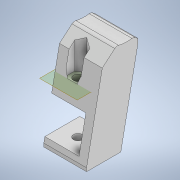
# Autodesk Inventor part: IntakeStop
Saved by Autodesk Inventor 2020 (Build 240168000, 168)
## iProperties
Created: 2020-02-14
Part Number: IntakeStop
Material: Generic
Document SubType Name: Modeling
Designer: srini
Density: 1 g/cm^3
Appearance: Default
Author: srini
Autodesk Inventor part; units mm, degrees
ref_plane "YZ Plane" through (0, 0, 0) normal (1, 0, 0) x (0, 1, 0)
ref_plane "XZ Plane" through (0, 0, 0) normal (0, 1, 0) x (-1, 0, 0)
ref_plane "XY Plane" through (0, 0, 0) normal (0, 0, 1) x (1, 0, 0)
sketch "Sketch1" plane through (0, 0, 0) normal (0, 0, 1) x (1, 0, 0)
  line L0 (15.875, -34.925) -> (-15.875, -34.925)
  line L1 (-15.875, -34.925) -> (-15.875, 34.925)
  line L2 (-15.875, 34.925) -> (15.875, 34.925)
  line L3 (15.875, 34.925) -> (15.875, -34.925)
  line L4 (15.875, -34.925) -> (-15.875, 34.925) construction
  line L5 (-15.875, -34.925) -> (15.875, 34.925) construction
  point P0 (0, 0)
  dimension "d0" = 31.75
  dimension "d1" = 69.85
  constraints: 12 end point, 2 midpoint, 2 parallel, 1 horizontal, 1 perpendicular
  measures "d0" distance of L1.end L2.end
  measures "d1" distance of L2.end L0.start
extrude "Extrusion1" add sketch "Sketch1" along normal blind 38.1
sketch "Sketch2" plane through (0, 0, 38.1) normal (0, 0, 1) x (1, 0, 0)
  line L0 (9.525, -28.575) -> (-15.875, -28.575)
  line L1 (-15.875, -28.575) -> (-15.875, -3.175)
  line L2 (-15.875, -3.175) -> (9.525, -3.175)
  line L3 (9.525, -3.175) -> (9.525, -28.575)
  line L4 (-15.875, -34.925) -> (15.875, -34.925) projected
  line L5 (15.875, -34.925) -> (15.875, 34.925) projected
  line L6 (-15.875, 34.925) -> (-15.875, -34.925) projected
  point P0 (0, 0)
  dimension "d4" = 6.35
  dimension "d5" = 6.35
  dimension "d6" = 25.4
  dimension "d7" = 25.4
  constraints: 8 end point, 2 parallel, 1 collinear, 1 horizontal, 1 perpendicular
  measures "d4" distance between parallel lines of L0 L4
  measures "d5" distance between parallel lines of L3 L5
  measures "d6" distance of L2.end L0.start
  measures "d7" distance of L0.start L0.end
extrude "Extrusion2" cut sketch "Sketch2" against normal through all
sketch "Sketch3" plane through (15.875, -34.925, 0) normal (1, 0, 0) x (0, 0, -1)
  line L0 (-38.1, 69.85) -> (-38.1, 31.75) projected
  line L1 (-38.1, 50.8) -> (-15.875, 69.85)
  line L2 (0, 69.85) -> (-38.1, 69.85) projected
  line L3 (-38.1, 50.8) -> (-38.1, 69.85)
  line L4 (-38.1, 69.85) -> (-15.875, 69.85)
  line L5 (0, 0) -> (0, 69.85) projected
  arc A0 (-15.875, 69.85) -> (0, 69.85) centre (-7.9375, 93.9779) ccw
  line L6 (0, 69.85) -> (-38.1, 69.85) projected
  line L7 (-15.875, 69.85) -> (0, 69.85)
  point P0 (0, 34.925)
  dimension "d10" = 15.875
  dimension "d11" = 19.05
  dimension "d23" = 25.4
  constraints: 8 end point, 2 point on circle, 1 centre point, 1 horizontal, 1 midpoint, 1 perpendicular, 1 point on line, 1 vertical
  measures "d10" distance of L2.start L1.end
  measures "d11" distance of L0.start L1.start
  measures "d23" radius of A0
extrude "Extrusion3" cut sketch "Sketch3" against normal through all
sketch "Sketch4" plane through (-15.875, -34.925, 0) normal (0, -1, 0) x (1, 0, 0)
  circle A0 centre (12.7, 25.4) radius 3.3734
  line L0 (0, 0) -> (0, 38.1) projected
  line L1 (0, 38.1) -> (31.75, 38.1) projected
  point P0 (15.875, 0)
  dimension "d14" = 12.7
  dimension "d15" = 12.7
  dimension "d16" = 6.7469
  constraints: 1 centre point
  measures "d14" distance from line of A0.centre L0
  measures "d15" distance from line of A0.centre L1
  measures "d16" diameter of A0
extrude "Extrusion4" cut sketch "Sketch4" against normal through all
ref_plane "Work Plane1" through (-15.875, 9.525, 38.1) normal (0, -1, 0) x (1, 0, 0)
sketch "Sketch5" plane through (-15.875, 9.525, 38.1) normal (0, -1, 0) x (1, 0, 0)
  circle A0 centre (12.7, -12.7) radius 3.3734 projected
  line L0 (7.1437, -9.4921) -> (12.7, -6.2842)
  line L1 (12.7, -6.2842) -> (18.2563, -9.4921)
  line L2 (18.2563, -9.4921) -> (18.2562, -15.9079)
  line L3 (18.2562, -15.9079) -> (12.7, -19.1158)
  line L4 (12.7, -19.1158) -> (7.1437, -15.9079)
  line L5 (7.1437, -15.9079) -> (7.1437, -9.4921)
  point P0 (15.875, -38.1)
  dimension "d20" = 11.1125
  constraints: 12 end point, 1 coincident, 1 vertical, 13 other
  measures "d20" distance between parallel lines of L2 L5
extrude "Extrusion5" cut sketch "Sketch5" against normal blind 38.1 contours A0 | L0 L1 L2 L3 L4 L5
fillet "Fillet1" radius 3.175 1 edges at (0, 34.925, 15.875)
chamfer "Chamfer1" distance 3.175 angle 45 1 edges at (0, 34.925, 0)
fillet "Fillet2" radius 3.175 1 edges at (0, 34.1233, 3.0721)
sketch "Sketch6" plane through (15.875, -34.925, 38.1) normal (1, 0, 0) x (0, 0, -1)
  line L0 (25.4, 0) -> (38.1, 63.5)
  line L1 (38.1, 63.5) -> (38.1, 0)
  line L2 (38.1, 0) -> (25.4, 0)
  line L3 (38.1, 0) -> (0, 0) projected
  line L4 (38.1, 0) -> (38.1, 66.675) projected
  line L5 (-4.7298, -21.134) -> (20.7966, 106.498)
  line L6 (20.7966, 106.498) -> (-6.997, 112.0567)
  line L7 (-6.997, 112.0567) -> (-32.5234, -15.5753)
  line L8 (-32.5234, -15.5753) -> (-4.7298, -21.134)
  point P0 (38.1, 34.925)
  dimension "d29" = 63.5
  dimension "d30" = 12.7
  dimension "d33" = 25.4
  constraints: 14 end point, 3 parallel, 2 collinear, 1 perpendicular
  measures "d29" distance of L0.end L1.end
  measures "d30" distance of L1.end L0.start
  measures "d33" distance between parallel lines of L0 L5
extrude "Extrusion6" cut sketch "Sketch6" against normal through all
body "Solid1"
